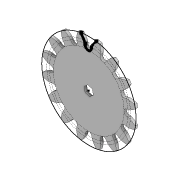
# Autodesk Inventor part: spruegear-module2-z16
Saved by Autodesk Inventor 2020 (Build 240168000, 168)
## iProperties
Created: 2021-06-14
Part Number: spruegear-module2-z16
Material: Generic
Document SubType Name: Modeling
Designer: Aidan Lee
Density: 1 g/cm^3
Appearance: Default
Author: Aidan Lee
Autodesk Inventor part; units mm, degrees
ref_plane "YZ Plane" through (0, 0, 0) normal (1, 0, 0) x (0, 1, 0)
ref_plane "XZ Plane" through (0, 0, 0) normal (0, 1, 0) x (-1, 0, 0)
ref_plane "XY Plane" through (0, 0, 0) normal (0, 0, 1) x (1, 0, 0)
sketch "Sketch1" plane through (0, 0, 0) normal (0, 0, 1) x (1, 0, 0)
  spline S0 degree 3 poles (-8.9262, 55.5372) (-8.7839, 55.3802) (-8.4991, 55.0662) (-8.0852, 54.5835) (-7.6813, 54.0924) (-7.2889, 53.592) (-6.9084, 53.0826) (-6.5406, 52.5638) (-6.1865, 52.0357) (-5.8469, 51.4981) (-5.5231, 50.9508) (-5.2164, 50.3937) (-4.9286, 49.8267) (-4.6617, 49.2495) (-4.4187, 48.6617) (-4.2033, 48.0633) (-4.0539, 47.5547) (-3.9553, 47.1422) (-3.9241, 46.9325) (-3.9085, 46.8277) knots 0 0 0 0 0.063581 0.127162 0.190743 0.254324 0.317905 0.381486 0.445066 0.508647 0.572227 0.635807 0.699386 0.762964 0.826542 0.890117 0.953687 0.985476 1.017256 1.017256 1.017256 1.017256
  spline S1 degree 3 poles (-3.9085, 46.8277) (-3.8988, 46.6849) (-3.8795, 46.3993) (-3.8286, 45.9728) (-3.7545, 45.5498) (-3.6583, 45.1311) (-3.5319, 44.7205) (-3.3763, 44.3201) (-3.189, 43.9333) (-2.9645, 43.5666) (-2.7433, 43.2845) (-2.5493, 43.0739) (-2.3922, 42.9274) (-2.2262, 42.7911) (-2.0526, 42.6646) (-1.8686, 42.5537) (-1.678, 42.4548) (-1.4812, 42.3683) (-1.2769, 42.302) (-1.0697, 42.2449) (-0.8577, 42.21) (-0.6441, 42.187) (-0.3577, 42.1846) (0, 42.1894) (0.3577, 42.1846) (0.6441, 42.187) (0.8577, 42.21) (1.0697, 42.2449) (1.2769, 42.302) (1.4812, 42.3683) (1.678, 42.4548) (1.8686, 42.5537) (2.0526, 42.6646) (2.2262, 42.7911) (2.3922, 42.9274) (2.5493, 43.0739) (2.7433, 43.2845) (2.9645, 43.5666) (3.189, 43.9333) (3.3763, 44.3201) (3.5319, 44.7205) (3.6583, 45.1311) (3.7545, 45.5498) (3.8286, 45.9728) (3.8795, 46.3993) (3.8988, 46.6849) (3.9085, 46.8277) knots 0 0 0 0 0.04293 0.085861 0.12879 0.17172 0.214646 0.257562 0.300476 0.343394 0.386302 0.407769 0.429238 0.450698 0.472163 0.49363 0.515088 0.536554 0.558017 0.579478 0.600945 0.622403 0.64387 0.686802 0.729734 0.751201 0.772659 0.794126 0.815587 0.83705 0.858516 0.879974 0.901441 0.922906 0.944366 0.965835 0.987302 1.03021 1.073128 1.116042 1.158958 1.201884 1.244814 1.287743 1.330674 1.373604 1.373604 1.373604 1.373604
  spline S2 degree 3 poles (3.9085, 46.8277) (3.9241, 46.9325) (3.9553, 47.1422) (4.0539, 47.5547) (4.2033, 48.0633) (4.4187, 48.6617) (4.6617, 49.2495) (4.9286, 49.8267) (5.2164, 50.3937) (5.5231, 50.9508) (5.8469, 51.4981) (6.1865, 52.0357) (6.5406, 52.5638) (6.9084, 53.0826) (7.2889, 53.592) (7.6813, 54.0924) (8.0852, 54.5835) (8.4991, 55.0662) (8.7839, 55.3802) (8.9262, 55.5372) knots 0 0 0 0 0.03178 0.063568 0.127139 0.190714 0.254291 0.31787 0.381449 0.445029 0.508609 0.572189 0.63577 0.699351 0.762932 0.826513 0.890094 0.953675 1.017256 1.017256 1.017256 1.017256
  circle A0 centre (0, 0) radius 42.1875 construction
  circle A1 centre (0, 0) radius 46.9846 construction
  circle A2 centre (0, 0) radius 50 construction
  circle A3 centre (0, 0) radius 56.25
  point P0 (-8.5013, 55.0643)
  point P1 (-8.0869, 54.5821)
  point P2 (-7.6832, 54.0908)
  point P3 (-7.2909, 53.5905)
  point P4 (-6.9105, 53.081)
  point P5 (-6.5429, 52.5623)
  point P6 (-6.1889, 52.0341)
  point P7 (-5.8496, 51.4965)
  point P8 (-5.526, 50.9492)
  point P9 (-5.2196, 50.3921)
  point P10 (-4.9321, 49.825)
  point P11 (-4.6657, 49.2477)
  point P12 (-4.4233, 48.6599)
  point P13 (-4.2093, 48.0613)
  point P14 (-4.031, 47.4511)
  point P15 (-3.9598, 47.1413)
  point P16 (-3.8758, 46.3996)
  point P17 (-3.8247, 45.9733)
  point P18 (-3.7508, 45.5505)
  point P19 (-3.6533, 45.1324)
  point P20 (-3.527, 44.7221)
  point P21 (-3.371, 44.3223)
  point P22 (-3.1828, 43.9367)
  point P23 (-2.9576, 43.5713)
  point P24 (-2.6935, 43.2332)
  point P25 (-2.5474, 43.0758)
  point P26 (-2.3907, 42.9291)
  point P27 (-2.225, 42.7928)
  point P28 (-2.0509, 42.6672)
  point P29 (-1.8675, 42.5557)
  point P30 (-1.677, 42.4569)
  point P31 (-1.48, 42.3717)
  point P32 (-1.2764, 42.3036)
  point P33 (-1.069, 42.2486)
  point P34 (-0.8574, 42.212)
  point P35 (-0.6439, 42.1905)
  point P36 (-0.4293, 42.1857)
  point P37 (0, 42.1875)
  point P38 (0.4293, 42.1857)
  point P39 (0.6439, 42.1905)
  point P40 (0.8574, 42.212)
  point P41 (1.069, 42.2486)
  point P42 (1.2764, 42.3036)
  point P43 (1.48, 42.3717)
  point P44 (1.677, 42.4569)
  point P45 (1.8675, 42.5557)
  point P46 (2.0509, 42.6672)
  point P47 (2.225, 42.7928)
  point P48 (2.3907, 42.9291)
  point P49 (2.5474, 43.0758)
  point P50 (2.6935, 43.2332)
  point P51 (2.9576, 43.5713)
  point P52 (3.1828, 43.9367)
  point P53 (3.371, 44.3223)
  point P54 (3.527, 44.7221)
  point P55 (3.6533, 45.1324)
  point P56 (3.7508, 45.5505)
  point P57 (3.8247, 45.9733)
  point P58 (3.8758, 46.3996)
  point P59 (3.9598, 47.1413)
  point P60 (4.031, 47.4511)
  point P61 (4.2093, 48.0613)
  point P62 (4.4233, 48.6599)
  point P63 (4.6657, 49.2477)
  point P64 (4.9321, 49.825)
  point P65 (5.2196, 50.3921)
  point P66 (5.526, 50.9492)
  point P67 (5.8496, 51.4965)
  point P68 (6.1889, 52.0341)
  point P69 (6.5429, 52.5623)
  point P70 (6.9105, 53.081)
  point P71 (7.2909, 53.5905)
  point P72 (7.6832, 54.0908)
  point P73 (8.0869, 54.5821)
  point P74 (8.5013, 55.0643)
  constraints: 4 centre point, 2 point on circle, 165 other
extrude "Extrusion1" add sketch "Sketch1" against normal blind 3
extrude "Extrusion2" cut sketch "Sketch1" against normal through all contours A3 S2 S1 S0 picked at (0.9155, 51.5438)
pattern_circular "Circular Pattern1" count 16 over 360 about axis through (0, 0, 0) along (0, 0, -1) of "Extrusion2"
sketch "Sketch2" plane through (0, 0, 0) normal (0, 0, 1) x (1, 0, 0)
  circle A0 centre (0, 0) radius 50 construction
  circle A1 centre (49.0393, 9.7545) radius 2.75
  arc A2 (55.5372, 8.9262) -> (54.7256, 13.0064) centre (0, 0) ccw projected
  line L0 (54.7256, 13.0064) -> (55.5372, 8.9262)
  line L1 (55.1314, 10.9663) -> (0, 0)
  circle A3 centre (0, 0) radius 56.25 projected
  line L2 (-5.4671, 1.8558) -> (-1.1264, 5.6626)
  line L3 (-1.1264, 5.6626) -> (4.3407, 3.8067)
  line L4 (4.3407, 3.8067) -> (5.4671, -1.8558)
  line L5 (5.4671, -1.8558) -> (1.1264, -5.6626)
  line L6 (1.1264, -5.6626) -> (-4.3407, -3.8067)
  line L7 (-4.3407, -3.8067) -> (-5.4671, 1.8558)
  point P0 (46.8277, 3.9085)
  point P1 (44.7588, 14.3092)
  dimension "d14" = 5.5
  dimension "d16" = 6.25
  dimension "d17" = 10
  constraints: 16 end point, 2 perpendicular, 1 centre point, 1 coincident, 1 midpoint, 1 point on line, 17 other
  measures "d14" diameter of A1
  measures "d17" distance between parallel lines of L2 L5
extrude "Extrusion3" cut sketch "Sketch2" against normal through all contours L4 L5 L6 L7 L2 L3
equation "\"Module\" = 6.25"
equation "\"PressureAngle\" = 20deg"
equation "\"UnitProfileClearance\" = 0.25"
equation "\"UnitRoundRadius\" = 0.35"
equation "\"HeadDiameter\" = 112.5"
equation "\"RootDiameter\" = 84.375"
equation "\"BaseDiameter\" = 93.96926"
equation "\"HelixAngle\" = 0"
equation "\"UnitCorrection\" = 0"
equation "\"UnitAddendumModification\" = 0"
equation "\"CircularPitch\" = 19.634954"
equation "\"UnitBacklashShift\" = 0"
equation "\"TotalToolShift\" = 0"
equation "\"IsInternal\" = 0"
body "Solid1"
